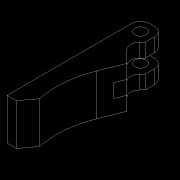
# Autodesk Inventor part: ProximalPhalangeIndex2
Saved by Autodesk Inventor 2015 (Build 190159000, 159)
## iProperties
Created: 2014-10-27
Part Number: ProximalPhalangeIndex2
Material: Generic
Document SubType Name: Modeling
Designer: Inventor
Mass: 0.970494 g
Surface Area: 9.37811 cm^2
Volume: 0.970494 cm^3
Density: 1 g/cm^3
Appearance: Default
RuleStatus: InUse
BeforeDocSave0: UpdateBoundingBox
CX: 7.00 mm
CY: 29.00 mm
CZ: 9.00 mm
Author: Inventor
Autodesk Inventor part; units mm, degrees
ref_plane "YZ Plane" through (0, 0, 0) normal (1, 0, 0) x (0, 1, 0)
ref_plane "XZ Plane" through (0, 0, 0) normal (0, 1, 0) x (-1, 0, 0)
sketch "Base" plane through (0, 0, 0) normal (0, 0, 1) x (1, 0, 0)
  line L0 (0, 0) -> (0, -29)
  line L1 (0, 0) -> (5, 0)
  line L2 (5, 0) -> (5, -4)
  line L3 (3, -6) -> (7, -10)
  line L4 (7, -10) -> (5.1554, -14.6473)
  line L5 (0, -29) -> (5, -29)
  line L6 (5, -4) -> (3, -6)
  arc A0 (5.1554, -14.6473) -> (5, -29) centre (23.7446, -22.0257) ccw
  dimension "d0" = 29
  dimension "d1" = 5
  dimension "d54" = 4
  dimension "d112" = 5
  dimension "d116" = 20
  dimension "d117" = 45
  dimension "d118" = 7
  dimension "d119" = 5
  dimension "d123" = 4
  constraints: 14 end point, 2 horizontal, 2 perpendicular, 2 point on circle, 1 centre point, 1 coincident, 1 tangent, 1 vertical
  measures "d0" distance of L0.start L0.end
  measures "d1" distance of L0.start L1.end
  measures "d54" distance of L1.end L2.end
  measures "d112" distance of L0.end L5.end
  measures "d116" radius of A0
  measures "d117" angle of L0 L3
  measures "d118" distance from line of L0 L3.end
  measures "d119" distance of L3.end L4.end
  measures "d123" horizontal distance of L3.start L3.end
extrude "BaseFeature" add sketch "Base" along normal blind 9
chamfer "EndChamferFeature" distance 3 angle 45 1 edges at (5, -29, 4.5)
sketch "MountHole" plane through (0, 0, 9) normal (0, 0, 1) x (1, 0, 0)
  circle A0 centre (2.5, -2.5) radius 1.25
  line L0 (5, 0) -> (0, 0) construction
  line L1 (0, 0) -> (0, -29) construction
  dimension "d40" = 2.5
  dimension "d41" = 2.5
  dimension "d42" = 2.5
  constraints: 1 centre point
  measures "d40" diameter of A0
  measures "d41" distance from line of L0 A0.centre
  measures "d42" distance from line of L1 A0.centre
hole "MountHoleFeature" at (2.5, -2.5, 9) direction (0, 0, -1) diameter 2.5 end through all
fillet "EndFilletsFeature" radius 2 2 edges at (0, 0, 4.5) (5, 0, 4.5)
ref_plane "MidPlane" through (0, 0, 4.5) normal (0, 0, 1) x (1, 0, 0)
sketch "MountCut" plane through (0, 0, 4.5) normal (0, 0, 1) x (1, 0, 0)
  line L0 (5.1554, -14.6473) -> (7, -10) projected
  line L1 (7, -10) -> (3, -6) projected
  line L2 (3, -6) -> (5, -4) projected
  arc A0 (5, -2) -> (3, 0) centre (3, -2) ccw projected
  line L3 (3, 0) -> (2, 0) projected
  arc A1 (2, 0) -> (0, -2) centre (2, -2) ccw projected
  line L4 (0, -2) -> (0, -29) projected
  circle A2 centre (2.5, -2.5) radius 1.25 projected
  line L5 (4.1677, -26.1178) -> (2, -29) projected
  arc A3 (5.1554, -14.6473) -> (4.1677, -26.1178) centre (23.7446, -22.0257) ccw projected
  line L6 (3, -6) -> (0, -6)
  line L7 (0, -12) -> (6.2062, -12)
  line L8 (5.1554, -14.6473) -> (7, -10) projected
  line L9 (0, -2) -> (0, -29) projected
  line L10 (0, -29) -> (2, -29) projected
  line L11 (5, -4) -> (5, -2) projected
  dimension "d120" = 6
  constraints: 4 end point, 3 point on line, 1 horizontal, 1 perpendicular
  measures "d120" distance between parallel lines of L6 L7
extrude "MountCutFeature" cut sketch "MountCut" along normal mid plane 3 contours L7 L4 L6 L1 L0 | L6 L4 A1 L3 A0 L11 L2
fillet "LastFilletFeature" radius 2 2 edges at (3, -6, 1.5) (3, -6, 7.5)
